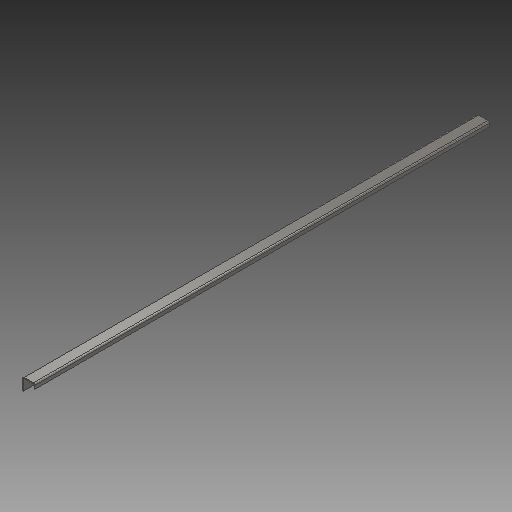
# Autodesk Inventor part: Perfil "J"
Saved by Autodesk Inventor 2017 (Build 210142000, 142)
## iProperties
Created: 2019-06-18
Part Number: Perfil "J"
Material: Stainless Steel
Description: Chapa de Aço Inox Aisi 304 - #1,5mm
Document SubType Name: Sheet Metal
Designer: leonardo.prado
Mass: 614.565 g
Surface Area: 1053.83 cm^2
Volume: 76.8207 cm^3
Density: 8 g/cm^3
Flat Pattern Width: 5.47858 cm
Flat Pattern Length: 93 cm
Flat Pattern Area: 509.508 cm^2
Sheet Metal Rule: Default_mm
Sheet Metal Width: 54,786 mm
Sheet Metal Length: 930,000 mm
Sheet Metal Area: 50950,831 mm^2
Appearance: Semi-Polished
Author: leonardo.prado
Comments: 55 x 930
Autodesk Inventor part; units mm, degrees
note: some values were not read from the file. Chosen so that the rebuilt part matches the saved one: flange form of "Plate1".
ref_plane "YZ Plane" through (0, 0, 0) normal (1, 0, 0) x (0, 1, 0)
ref_plane "XZ Plane" through (0, 0, 0) normal (0, 1, 0) x (-1, 0, 0)
ref_plane "XY Plane" through (0, 0, 0) normal (0, 0, 1) x (1, 0, 0)
sketch "Sketch1" plane through (0, 0, 0) normal (0, 0, 1) x (1, 0, 0)
  line L0 (0, 0) -> (0, 25)
  line L1 (0, 25) -> (25, 25)
  line L2 (25, 25) -> (25, 15)
  dimension "d0" = 25
  dimension "d1" = 25
  dimension "d2" = 10
  measures "d0" distance of L0.start L0.end
  measures "d1" distance of L0.end L1.end
  measures "d2" distance of L1.end L2.end
contour flange "Contour Flange1" sketch "Sketch1" thickness 1.5 bend radius 1.5 width 930 along (0, 0, 1) mid plane yes both sides no wall seen from (0, 12.5, 0) lies toward (1, 0, 0) curves L0 L1 L2
bend "Bend1"
corner "Corner1"
equation "\"d3\" = BendReliefWidth"
equation "\"d4\" = BendReliefDepth"
equation "\"d5\" = MinimumRemnant"
equation "\"d6\" = BendRadius"
equation "\"d8\" = BendRadius"
equation "\"d10\" = CornerReliefSize"
equation "\"d11\" = GapSize"
equation "\"d12\" = JacobiRadiusSize"
equation "\"BendRadius\" = Thickness"
equation "\"BendReliefWidth\" = Thickness"
equation "\"BendReliefDepth\" = 0.5 * Thickness"
equation "\"CornerReliefSize\" = 4 * Thickness"
equation "\"MinimumRemnant\" = 2 * Thickness"
equation "\"TransitionRadius\" = BendRadius"
equation "\"JacobiRadiusSize\" = BendRadius"
equation "\"GapSize\" = Thickness"
equation "\"Thickness\" = 1.5"
body "Solid1"
